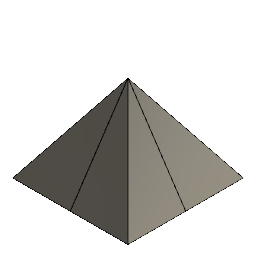
Pyramid v2 (Autodesk Fusion 360 design; units mm, degrees)
Autodesk Fusion 360 part; units mm, degrees
sketch "Sketch1" plane through (0, 0, 0) normal (0, 0, 1) x (1, 0, 0)
  circle A0 centre (0, 0) radius 5
  constraint coincident A0.centre origin
sketch "Sketch2" plane through (0, 0, 0) normal (0, 0, 1) x (1, 0, 0)
  line L0 (0, 0) -> (10, 0)
  line L1 (10, 0) -> (10, 10)
  line L2 (10, 10) -> (0, 10)
  line L3 (0, 10) -> (0, 0)
  constraint horizontal L0
  constraint vertical L1
  constraint horizontal L2
  constraint vertical L3
  constraint coincident L0.start L3.end
form "Form1" [no effect]
sketch "sketch 927" plane through (0, 0, 0) normal (0, 0, 1) x (1, 0, 0)
  line L0 (0, 0) -> (10, 0)
  line L1 (10, 0) -> (10, 10)
  line L2 (10, 10) -> (0, 10)
  line L3 (0, 10) -> (0, 0)
  constraint horizontal L0
  constraint vertical L1
  constraint horizontal L2
  constraint vertical L3
  constraint coincident L0.start L3.end
extrude "Extrude3" add sketch "sketch 927" along normal blind 10 makes body 1
form "Form2" [no effect]
chamfer "Chamfer1" distance 9.999 angle 45 2 edges at (5, 10, 10) (0, 5, 10) on bodies 1
copy_body "CopyPasteBodies1" bodies 1 makes body 2
move_body "Move1" bodies 2 to x (1, 0, 0) y (0, 1, 0) z (0, 0, 1) at (10, 0, 0)
copy_body "CopyPasteBodies2" bodies 1 2 makes body 3 makes body 4
move_body "Move2" bodies 3 4 to x (1, 0, 0) y (0, 1, 0) z (0, 0, 1) at (0, -10, 0)
move_body "Move3" bodies 3 to x (0, 1, 0) y (-1, 0, 0) z (0, 0, 1) at (0, -10, 0)
move_body "Move4" bodies 2 to x (0, -1, 0) y (1, 0, 0) z (0, 0, 1) at (10, 20, 0)
move_body "Move5" bodies 4 to x (-1, 0, 0) y (0, -1, 0) z (0, 0, 1) at (30, -10, 0)
scale "Scale1" factors (1, 1, 1.5) about (9.999, -0.001, 10) bodies 1 2 4 3
scale "Scale2" factor 0.5 about (10, -0.001, 10) bodies 1 3 2 4
